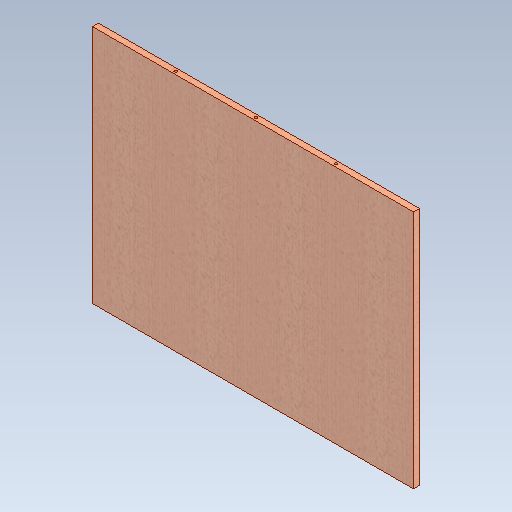
# Autodesk Inventor part: LateralMayor
Saved by Autodesk Inventor 2020.3 (Build 243373000, 373)
## iProperties
Created: 2020-10-27
Part Number: LateralMayor
Material: Madera (roble)
Document SubType Name: Modeling
Designer: codig
Density: 0.76 g/cm^3
Appearance: Roble blanco - Natural brillo medio
Author: codig
Autodesk Inventor part; units mm, degrees
ref_plane "YZ Plane" through (0, 0, 0) normal (1, 0, 0) x (0, 1, 0)
ref_plane "XZ Plane" through (0, 0, 0) normal (0, 1, 0) x (-1, 0, 0)
ref_plane "XY Plane" through (0, 0, 0) normal (0, 0, 1) x (1, 0, 0)
sketch "Boceto1" plane through (0, 0, 0) normal (0, 0, 1) x (1, 0, 0)
  line L0 (100, 100) -> (1064, 100)
  line L1 (1064, 100) -> (1064, 820)
  line L2 (1064, 820) -> (100, 820)
  line L3 (100, 820) -> (100, 100)
  point P0 (0, 0)
  constraints: 8 end point, 2 parallel, 1 horizontal, 1 perpendicular
extrude "Extrusión1" add sketch "Boceto1" along normal blind 18
sketch "Boceto2" plane through (100, 820, 0) normal (0, 1, 0) x (1, 0, 0)
  line L0 (964, 0) -> (964, -18) projected
  line L1 (964, 0) -> (0, 0) projected
  circle A0 centre (241, -9) radius 4
  circle A1 centre (482, -9) radius 4
  circle A2 centre (723, -9) radius 4
  point P0 (-100, 0)
  constraints: 3 centre point
hole "Agujero1" at (341, 820, 9) at (582, 820, 9) at (823, 820, 9) direction (0, -1, 0) diameter 8 depth 35
sketch "Boceto3" plane through (0, 0, 0) normal (0, 0, -1) x (-1, 0, 0)
  line L0 (-100, 100) -> (-1064, 100) projected
  circle A0 centre (-109, 640) radius 4
  circle A1 centre (-109, 460) radius 4
  circle A2 centre (-109, 280) radius 4
  point P0 (0, 0)
  constraints: 3 centre point
hole "Agujero2" at (109, 640, 0) at (109, 460, 0) at (109, 280, 0) direction (0, 0, 1) diameter 8 depth 10
sketch "Boceto5" plane through (0, 0, 0) normal (0, 0, -1) x (-1, 0, 0)
  circle A0 centre (-954, 321) radius 4
  line L0 (-1064, 100) -> (-1064, 820) projected
  circle A1 centre (-844, 321) radius 4
  circle A2 centre (-734, 321) radius 4
  point P0 (0, 0)
  constraints: 3 centre point
hole "Agujero4" at (954, 321, 0) at (844, 321, 0) at (734, 321, 0) direction (0, 0, 1) diameter 8 depth 10
sketch "Boceto8" plane through (0, 0, 0) normal (0, 0, -1) x (-1, 0, 0)
  circle A0 centre (-954, 129) radius 4
  circle A1 centre (-844, 129) radius 4
  circle A2 centre (-734, 129) radius 4
  point P0 (0, 0)
  constraints: 3 centre point
hole "Agujero5" at (954, 129, 0) at (844, 129, 0) at (734, 129, 0) direction (0, 0, 1) diameter 8 depth 10
sketch "Boceto9" plane through (100, 100, 0) normal (0, -1, 0) x (1, 0, 0)
  circle A0 centre (241, 9) radius 4 projected
  circle A1 centre (241, 9) radius 4
  circle A2 centre (482, 9) radius 4 projected
  circle A3 centre (482, 9) radius 4
  circle A4 centre (723, 9) radius 4 projected
  circle A5 centre (723, 9) radius 4
  point P0 (-100, 0)
  constraints: 3 centre point, 3 coincident
hole "Agujero6" at (341, 100, 9) at (582, 100, 9) at (823, 100, 9) direction (0, 1, 0) diameter 8 depth 23
